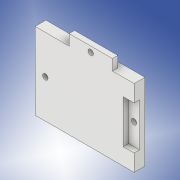
# Autodesk Inventor part: SP005
Saved by Autodesk Inventor 2017 SP1 (Build 210196100, 196)
## iProperties
Created: 2017-08-09
Part Number: SP005
Material: ABS Plastic
Document SubType Name: Modeling
Designer: Zach
Density: 1.06 g/cm^3
Appearance: CR White
Author: Zach
Autodesk Inventor part; units mm, degrees
ref_plane "YZ Plane" through (0, 0, 0) normal (1, 0, 0) x (0, 1, 0)
ref_plane "XZ Plane" through (0, 0, 0) normal (0, 1, 0) x (-1, 0, 0)
ref_plane "XY Plane" through (0, 0, 0) normal (0, 0, 1) x (1, 0, 0)
sketch "Sketch1" plane through (0, 0, 0) normal (0, 0, 1) x (1, 0, 0)
  line L0 (0, 0) -> (72.4, 0)
  line L1 (72.4, 0) -> (72.4, 71)
  line L2 (72.4, 71) -> (0, 71)
  line L3 (0, 71) -> (0, 0)
  dimension "d0" = 72.4
  dimension "d1" = 71
  constraints: 8 end point, 2 parallel, 1 horizontal, 1 perpendicular
  measures "d0" distance of L1.end L2.end
  measures "d1" distance of L0.end L1.end
extrude "Extrusion1" add sketch "Sketch1" along normal blind 10
sketch "Sketch2" plane through (0, 0, 10) normal (0, 0, 1) x (1, 0, 0)
  line L0 (72.4, 71) -> (0, 71) projected
  line L1 (52.4, 71) -> (12.4, 71)
  line L2 (12.4, 71) -> (12.4, 81)
  line L3 (12.4, 81) -> (52.4, 81)
  line L4 (52.4, 81) -> (52.4, 71)
  circle A0 centre (32.4, 76) radius 2.5
  line L5 (72.4, 0) -> (72.4, 71) projected
  point P0 (0, 0)
  point P1 (52.4, 76)
  point P2 (32.4, 81)
  dimension "d4" = 40
  dimension "d5" = 10
  dimension "d6" = 5
  dimension "d7" = 20
  constraints: 8 end point, 2 midpoint, 2 parallel, 1 centre point, 1 horizontal, 1 horizontal alignment, 1 perpendicular, 1 point on line, 1 vertical alignment
  measures "d4" distance of L2.end L3.end
  measures "d5" distance of L1.end L2.end
  measures "d6" diameter of A0
  measures "d7" distance between parallel lines of L5 L4
extrude "Extrusion2" add sketch "Sketch2" against normal blind 5
sketch "Sketch3" plane through (0, 0, 10) normal (0, 0, 1) x (1, 0, 0)
  line L0 (0, 71) -> (0, 0) projected
  line L1 (0, 0) -> (-19, 0)
  line L2 (-19, 0) -> (-19, 71)
  line L3 (-19, 71) -> (0, 71)
  line L4 (0, 71) -> (0, 0)
  line L5 (12.4, 71) -> (0, 71) projected
  circle A0 centre (-9.5, 35.5) radius 2.5
  point P0 (-19, 35.5)
  point P1 (-9.5, 71)
  dimension "d10" = 19
  dimension "d13" = 5
  constraints: 8 end point, 2 horizontal alignment, 2 midpoint, 2 parallel, 1 centre point, 1 horizontal, 1 perpendicular, 1 vertical alignment
  measures "d10" distance of L2.end L3.end
  measures "d13" diameter of A0
extrude "Extrusion3" add sketch "Sketch3" against normal blind 10
sketch "Sketch4" plane through (0, 0, 10) normal (0, 0, 1) x (1, 0, 0)
  line L0 (-19, 0) -> (72.4, 0) projected
  line L1 (52.4, 0) -> (12.4, 0)
  line L2 (12.4, 0) -> (12.4, 10)
  line L3 (12.4, 10) -> (52.4, 10)
  line L4 (52.4, 10) -> (52.4, 0)
  line L5 (72.4, 0) -> (72.4, 71) projected
  line L6 (72.4, 55.5) -> (62.4, 55.5)
  line L7 (62.4, 55.5) -> (62.4, 15.5)
  line L8 (62.4, 15.5) -> (72.4, 15.5)
  line L9 (72.4, 15.5) -> (72.4, 55.5)
  point P0 (0, 0)
  point P1 (72.4, 35.5)
  point P2 (72.4, 35.5)
  point P3 (52.4, 81)
  dimension "d16" = 40
  dimension "d17" = 10
  dimension "d18" = 10
  dimension "d19" = 40
  constraints: 16 end point, 4 parallel, 2 horizontal, 2 midpoint, 2 perpendicular, 2 point on line, 1 coincident, 1 vertical alignment
  measures "d16" distance of L2.end L3.end
  measures "d17" distance of L1.end L2.end
  measures "d18" distance of L8.end L7.end
  measures "d19" distance of L7.end L6.end
extrude "Extrusion4" cut sketch "Sketch4" against normal blind 5 contours L8 L7 L6 L5
sketch "Sketch5" plane through (0, 0, 5) normal (0, 0, 1) x (1, 0, 0)
  line L0 (62.4, 55.5) -> (72.4, 55.5) construction
  line L1 (62.4, 15.5) -> (62.4, 55.5) construction
  line L2 (72.4, 15.5) -> (62.4, 15.5) construction
  line L3 (72.4, 55.5) -> (72.4, 15.5) construction
  line L4 (52.4, 10) -> (52.4, 0) construction
  line L5 (12.4, 10) -> (52.4, 10) construction
  line L6 (12.4, 0) -> (12.4, 10) construction
  line L7 (52.4, 0) -> (12.4, 0) construction
  circle A0 centre (32.4, 5) radius 2.5
  circle A1 centre (67.4, 35.5) radius 2.5
  point P0 (0, 0)
  point P1 (62.4, 35.5)
  point P2 (12.4, 5)
  point P3 (67.4, 55.5)
  point P4 (32.4, 10)
  dimension "d22" = 5
  dimension "d23" = 5
  constraints: 4 midpoint, 2 centre point, 2 horizontal alignment, 2 vertical alignment
  measures "d22" diameter of A0
  measures "d23" diameter of A1
extrude "Extrusion5" cut sketch "Sketch5" against normal through all contours A1
body "Solid1"
